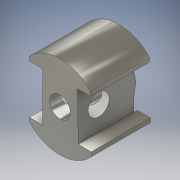
# Autodesk Inventor part: reverse gear cross head 1
Saved by Autodesk Inventor 2017 (Build 210142000, 142)
## iProperties
Created: 2018-10-31
Part Number: reverse gear cross head 1
Material: Generic
Document SubType Name: Modeling
Designer: User
Density: 1 g/cm^3
Appearance: Default
Author: User
Autodesk Inventor part; units mm, degrees
ref_plane "YZ Plane" through (0, 0, 0) normal (1, 0, 0) x (0, 1, 0)
ref_plane "XZ Plane" through (0, 0, 0) normal (0, 1, 0) x (-1, 0, 0)
ref_plane "XY Plane" through (0, 0, 0) normal (0, 0, 1) x (1, 0, 0)
sketch "Sketch1" plane through (0, 0, 0) normal (0, 1, 0) x (-1, 0, 0)
  circle A0 centre (0, 0) radius 12 construction
  line L0 (8.75, -7) -> (5, -7)
  line L1 (8.75, 7) -> (5, 7)
  line L2 (-5, 7) -> (-8.75, 7)
  line L3 (-5.25, -6.7253) -> (-9, -6.7253)
  line L4 (8.75, -7) -> (8.75, -8.212)
  line L5 (8.75, 7) -> (8.75, 8.212)
  line L6 (-8.75, 7) -> (-8.75, 8.212)
  arc A1 (8.75, 8.212) -> (-8.75, 8.212) centre (0, 0) ccw
  arc A2 (5, 7) -> (-5, 7) centre (0, 3.6834) ccw
  line L7 (-9, -6.7253) -> (-9, -7.9373)
  arc A3 (-9, -7.9373) -> (8.75, -8.212) centre (0, 0) ccw
  arc A4 (-5.25, -6.7253) -> (5, -7) centre (-0.0415, -3.7468) ccw
  circle A5 centre (0, 0) radius 4.75
  circle A6 centre (0, 0) radius 3
  line L8 (5, 7) -> (5, -7)
  line L9 (-5, 7) -> (-5.25, -6.7253)
  dimension "d0" = 24
  dimension "d2" = 3.75
  dimension "d3" = 3.75
  dimension "d5" = 3.75
  dimension "d6" = 3.75
  dimension "d28" = 8.75
  dimension "d29" = 14
  dimension "d31" = 1.212
  dimension "d32" = 1.212
  dimension "d33" = 6
  dimension "d34" = 1.212
  dimension "d35" = 1.212
  dimension "d49" = 9.5
  dimension "d50" = 6
  dimension "d51" = 1.044
  constraints: 20 end point, 12 point on circle, 7 centre point, 4 horizontal, 3 coincident, 3 equal radius, 3 vertical, 1 collinear, 1 parallel
  measures "d0" diameter of A0
  measures "d2" distance of L0.start L0.end
  measures "d3" distance of L1.start L1.end
  measures "d5" distance of L2.start L2.end
  measures "d6" distance of L3.start L3.end
  measures "d28" distance from line of point (0, 0) L4
  measures "d29" distance from line of L3.start L4
  measures "d31" distance of L1.start L5.end
  measures "d32" distance of L2.end L6.end
  measures "d33" radius of A2
  measures "d34" distance of L3.end L7.end
  measures "d35" distance of L0.start L4.end
  measures "d49" diameter of A5
  measures "d50" diameter of A6
  measures "d51" angle of L9 L5
extrude "Extrusion3" add sketch "Sketch1" along normal blind 16 contours A4 L9 A2 L8
extrude "Extrusion5" add sketch "Sketch1" along normal blind 17 contours L4 A3 L7 L3 A4 L0 | A2 L2 L6 A1 L5 L1 | A5
sketch "Sketch2" plane through (5.25, 0, -6.7253) normal (0.9998342, 0, 0.0182116) x (0.0182116, 0, -0.9998342)
  line L0 (-13.7275, 0) -> (0, 0) projected
  line L1 (0, 0) -> (0, 16) projected
  line L2 (-13.7275, 16) -> (0, 16) projected
  line L3 (-13.7275, 0) -> (-13.7275, 16) projected
  circle A0 centre (-6.8638, 6) radius 3
  line L4 (2.9272, 16) -> (0, 16) projected
  line L5 (0.0881, 0) -> (-13.9096, 0) projected
  line L6 (-13.9096, 0) -> (-13.9096, 16) projected
  line L7 (0.0881, 16) -> (-13.9096, 16) projected
  line L8 (0.0881, 0) -> (0.0881, 16) projected
  point P0 (-6.8197, 0)
  dimension "d54" = 6
  dimension "d55" = 6
  constraints: 1 centre point
  measures "d54" diameter of A0
  measures "d55" distance from line of L0 A0.centre
extrude "Extrusion6" cut sketch "Sketch2" against normal through all contours A0
fillet "Fillet1" radius 2 1 edges at (4.75, 16, 0)
body "Solid2"
